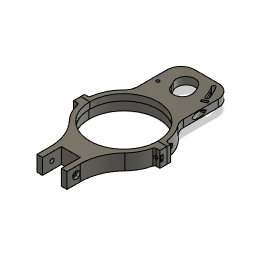
Generic Lens Mount and Focuser (Autodesk Fusion 360 design; units mm, degrees)
Autodesk Fusion 360 part; units mm, degrees
sketch "Sketch1" plane through (0, 0, 0) normal (0, 1, 0) x (1, 0, 0)
  circle A0 centre (0, 0) radius 37.25
  circle A1 centre (0, 0) radius 42.25
  line L0 (-37.25, 0) -> (37.25, 0) construction
  line L1 (-37.25, 0) -> (-42.25, 0)
  line L2 (37.25, 0) -> (42.25, 0)
  circle A2 centre (0.3022, 66.2) radius 21.95 construction
  circle A3 centre (-19.5912, 56.9235) radius 1.75
  arc A4 (11.2701, 65.1928) -> (6.5807, 75.2493) centre (-19.5912, 56.9235) ccw
  arc A5 (-8.0484, 60.0164) -> (11.2701, 65.1928) centre (1.6108, 62.6046) ccw
  arc A6 (-8.0484, 60.0164) -> (-9.8024, 63.7778) centre (-19.5912, 56.9235) ccw
  arc A7 (6.5807, 75.2493) -> (-9.8024, 63.7778) centre (-1.6108, 69.5135) ccw
  arc A8 (1.6108, 62.6046) -> (-1.6108, 69.5135) centre (-19.5912, 56.9235) ccw construction
  arc A9 (24.5033, 68.7386) -> (17.8031, 83.1073) centre (-19.5912, 56.9235) ccw
  arc A10 (21.1225, 67.8328) -> (24.5033, 68.7386) centre (22.8129, 68.2857) ccw
  arc A11 (21.1225, 67.8328) -> (14.936, 81.0998) centre (-19.5912, 56.9235) ccw
  arc A12 (17.8031, 83.1073) -> (14.936, 81.0998) centre (16.3695, 82.1035) ccw
  arc A13 (22.8129, 68.2857) -> (16.3695, 82.1035) centre (-19.5912, 56.9235) ccw construction
  line L3 (-19.5912, 56.9235) -> (16.3695, 82.1035) construction
  line L4 (-19.5912, 56.9235) -> (22.8129, 68.2857) construction
  line L5 (-25.3412, 33.8066) -> (-25.3412, 87.8535)
  line L6 (-25.3412, 87.8535) -> (30.5629, 87.8535)
  line L7 (0, 87.8535) -> (0, 0) construction
  circle A14 centre (0, 0) radius 38.25
  line L8 (16.3695, 82.1035) -> (22.8129, 68.2857)
  line L9 (-1.6108, 69.5135) -> (1.6108, 62.6046) construction
  line L10 (0, 66.0591) -> (1.6108, 62.6046)
  line L11 (-19.5912, 56.9235) -> (20.1957, 75.4765) construction
  line L12 (30.5629, 87.8535) -> (30.5629, 29.1714)
  line L13 (-42.25, 0) -> (-47.25, 0)
  line L14 (-47.25, 0) -> (-47.25, 4)
  line L15 (-47.25, 4) -> (-42.0602, 4)
  line L16 (47.25, 4) -> (42.0602, 4)
  line L17 (47.25, 0) -> (47.25, 4)
  line L18 (42.25, 0) -> (47.25, 0)
  line L19 (-47.25, 0) -> (-47.25, -7.85)
  line L20 (-47.25, -7.85) -> (-41.5143, -7.85)
  line L21 (47.25, 0) -> (47.25, -7.85)
  line L22 (47.25, -7.85) -> (41.5143, -7.85)
  line L23 (16.375, -38.9477) -> (16.375, -78.75)
  line L24 (16.375, -78.75) -> (10.375, -78.75)
  line L25 (10.375, -78.75) -> (10.375, -58)
  line L26 (10.375, -58) -> (-10.375, -58)
  line L27 (-10.375, -58) -> (-10.375, -78.75)
  line L28 (-10.375, -78.75) -> (-16.375, -78.75)
  line L29 (-16.375, -78.75) -> (-16.375, -38.9477)
  line L30 (0, 0) -> (0, -58)
  dimension "d1" = 74.5
  dimension "d2" = 5
  dimension "d3" = 43.9
  dimension "d4" = 3.5
  dimension "d5" = 10
  dimension "d7" = 1.75
  dimension "d8" = 20
  dimension "d11" = 5.75
  dimension "d14" = 76.5
  dimension "d26" = 65
  dimension "d28" = 5.75
  dimension "d29" = 7.75
  dimension "d57" = 5
  dimension "d58" = 4
  dimension "d59" = 7.85
  dimension "d94" = 66.2
  dimension "d99" = 6
  dimension "d100" = 6
  dimension "d101" = 20.75
  dimension "d102" = 20.75
  dimension "d123" = 58
  constraint coincident A0.centre A1.centre
  constraint coincident A0 L0.start
  constraint coincident A0 L0.end
  constraint coincident A0.centre L0
  constraint horizontal L0
  constraint coincident A1 L1.end
  constraint parallel L0 L1
  constraint coincident A1 L2.end
  constraint parallel L0 L2
  constraint coincident A2 A3.centre
  constraint tangent A4 A5
  constraint tangent A5 A6
  constraint tangent A6 A7
  constraint tangent A4 A7
  constraint coincident A3.centre A4.centre
  constraint coincident A2.centre A8
  constraint tangent A9 A10
  constraint tangent A10 A11
  constraint tangent A11 A12
  constraint tangent A9 A12
  constraint coincident A12.centre A13.end
  constraint coincident A10.centre A13.start
  constraint coincident A5.centre L4
  constraint coincident A7.centre L3
  constraint tangent A2 A13
  constraint coincident A1 L5.start
  constraint vertical L5
  constraint perpendicular L5 L6
  constraint vertical L7
  constraint concentric A0 A14
  constraint coincident A7.centre A8.end
  constraint coincident A5.centre A8.start
  constraint midpoint L9 L10.start
  constraint coincident L7 L10.start
  constraint midpoint A13 L11.end
  constraint coincident A2.centre L11
  constraint coincident A1 L12.end
  constraint perpendicular L6 L12
  constraint coincident L6 L7.start
  constraint parallel L1 L13
  constraint perpendicular L1 L14
  constraint coincident A1 L15.end
  constraint perpendicular L14 L15
  constraint symmetric L1.end L7 L2.end
  constraint symmetric L7 L13.end L17.start
  constraint symmetric L7 L14.end L16.start
  constraint symmetric L7 L15.end L16.end
  constraint perpendicular L13 L19
  constraint coincident A1 L20.end
  constraint perpendicular L19 L20
  constraint symmetric L7 L19.end L21.end
  constraint symmetric L7 L20.end L22.end
  constraint coincident A1 L23.start
  constraint vertical L23
  constraint perpendicular L23 L24
  constraint perpendicular L24 L25
  constraint perpendicular L25 L26
  constraint perpendicular L26 L27
  constraint perpendicular L27 L28
  constraint coincident A1 L29.end
  constraint perpendicular L28 L29
  constraint collinear L24 L28
  constraint midpoint L26 L30.end
  constraint vertical L30
  measures "d1" diameter of A0
  measures "d3" diameter of A2
  measures "d4" diameter of A3
  measures "d5" radius of A5
  measures "d7" radius of A10
  measures "d8" angle of L3 L4
  measures "d11" distance of A3.centre L5
  measures "d14" diameter of A14
  measures "d26" angle of L0 L8
  measures "d28" distance of A12.centre L6
  measures "d29" distance of A10.centre L12
  measures "d57" distance of L1.end L13.end
  measures "d58" distance of L13.end L14.end
  measures "d59" distance of L13.end L19.end
  measures "d94" vertical distance of A0.centre A2.centre
  measures "d99" distance of L23.end L24.end
  measures "d100" distance of L27.end L28.end
  measures "d101" distance of L25.end L26.end
  measures "d102" distance of L26.end L27.end
  measures "d123" distance of A0.centre L30.end
extrude "Extrude1" add sketch "Sketch1" along normal blind 7 contours A0 L1 L2 A14 | A1 L1 L2 A14 | A1 L16 L17 L18 | A1 L13 L14 L15 makes body 1
extrude "Extrude2" add sketch "Sketch1" against normal blind 10 contours A1 L1 L2 A14 | A1 L16 L17 L18 | A1 L13 L14 L15 bodies 1
extrude "Extrude3" add sketch "Sketch1" against normal blind 8 from surface at 7 contours A1 L5 L6 L12 bodies 1
extrude "Extrude4" add sketch "Sketch1" along normal blind 7 separate body contours A0 L2 A14 L30 | A0 L1 A14 L30 | A1 L2 A14 L30 | A1 L1 A14 L30 | A1 L18 L21 L22 | A1 L13 L19 L20 makes body 2
extrude "Extrude5" add sketch "Sketch1" against normal blind 10 contours A1 L2 A14 L30 | A1 L1 A14 L30 | A1 L18 L21 L22 | A1 L13 L19 L20 bodies 2
fillet "Fillet1" radius 15 2 edges at (-25.3412, 3, -87.8535) (30.5629, 3, -87.8535) on bodies 1
ref_plane "WorkPlane1" through (22.8129, 0, -68.2857) normal (0.422618, 0, 0.906308) x (0, 1, 0)
sketch "Sketch2" plane through (22.8129, 0, -68.2857) normal (0.422618, 0, 0.906308) x (0, 1, 0)
  line L0 (0, 0) -> (3, 0)
  circle A0 centre (3, 0) radius 1.75
  line L1 (4.7321, -3) -> (6.4641, 0) construction
  line L2 (6.4641, 0) -> (4.7321, 3) construction
  line L3 (4.7321, 3) -> (1.2679, 3)
  line L4 (1.2679, 3) -> (-0.4641, 0)
  line L5 (-0.4641, 0) -> (1.2679, -3)
  line L6 (1.2679, -3) -> (4.7321, -3)
  line L7 (3, 3) -> (7, 3)
  line L8 (7, 3) -> (7, -3)
  line L9 (3, -3) -> (7, -3)
  circle A1 centre (3, 0) radius 3.1
  point P0 (3, 0)
  dimension "d38" = 3.5
  dimension "d39" = 3
  dimension "d40" = 4
  dimension "d41" = 6.2
  dimension "d44" = 7
  constraint coincident L0.start origin
  constraint horizontal L0
  constraint coincident P0 L0.end
  constraint midpoint L3 L7.start
  constraint parallel L3 L7
  constraint perpendicular L3 L8
  constraint midpoint L6 L9.start
  constraint perpendicular L8 L9
  constraint concentric A0 A1
  constraint vertical L8
  measures "d38" diameter of A0
  measures "d39" distance of P0 L6
  measures "d40" distance of L9.start L8.end
  measures "d41" diameter of A1
  measures "d44" distance of L8 L0.start
extrude "Extrude6" cut sketch "Sketch2" along normal up to surface and the other way blind 15 contours A0 end surface through (30.5629, 7, -87.8535) normal (1, 0, 0) offset 0 bodies 1
extrude "Extrude7" cut sketch "Sketch2" along normal up to surface from surface at 10.5 contours L3 L4 L5 L6 L7 L9 A1 | L3 L7 A1 | L6 L9 A1 | L4 A1 | L5 A1 end surface through (30.5629, 7, -87.8535) normal (1, 0, 0) offset 0 bodies 1
extrude "Extrude8" cut sketch "Sketch2" along normal blind 2.65 from surface at 4 contours L3 L6 L7 L8 L9 A1 | L3 L4 L5 L6 L7 L9 A1 | L3 L4 A1 | L5 L6 A1 | L4 L5 A1 bodies 1
fillet "Fillet5" radius 2 2 edges at (-41.5143, -1.5, 7.85) (41.5143, -1.5, 7.85) on bodies 2
sketch "Sketch3" plane through (0, 0, -4) normal (0, 0, -1) x (-1, 0, 0)
  line L0 (47.25, -10) -> (47.25, 7)
  line L1 (47.25, 7) -> (42.0602, 7)
  line L2 (42.0602, 7) -> (42.0602, -10)
  line L3 (42.0602, -10) -> (47.25, -10)
  line L4 (47.25, -1.5) -> (43.25, -1.5) construction
  circle A0 centre (43.25, -1.5) radius 1.75
  circle A1 centre (43.25, -1.5) radius 3.1
  line L5 (44.9821, -4.5) -> (46.7141, -1.5) construction
  line L6 (46.7141, -1.5) -> (44.9821, 1.5) construction
  line L7 (44.9821, 1.5) -> (41.5179, 1.5)
  line L8 (41.5179, 1.5) -> (39.7859, -1.5)
  line L9 (39.7859, -1.5) -> (41.5179, -4.5)
  line L10 (41.5179, -4.5) -> (44.9821, -4.5)
  line L11 (44.9821, 1.5) -> (47.25, 1.5)
  line L12 (44.9821, -4.5) -> (47.25, -4.5)
  point P0 (43.25, -1.5)
  dimension "d60" = 4
  dimension "d61" = 3.5
  dimension "d62" = 6.2
  dimension "d63" = 3
  constraint midpoint L0 L4.start
  constraint perpendicular L2 L4
  constraint coincident P0 L4.end
  constraint concentric A0 A1
  constraint coincident L0 L11.end
  constraint perpendicular L0 L11
  constraint coincident L0 L12.end
  constraint perpendicular L0 L12
  constraint horizontal L10
  measures "d60" distance of L4.start P0
  measures "d61" diameter of A0
  measures "d62" diameter of A1
  measures "d63" distance of P0 L10
sketch "Sketch4" plane through (0, 0, -4) normal (0, 0, -1) x (-1, 0, 0)
  line L0 (-42.0602, -10) -> (-42.0602, 7)
  line L1 (-42.0602, 7) -> (-47.25, 7)
  line L2 (-47.25, 7) -> (-47.25, -10)
  line L3 (-47.25, -10) -> (-42.0602, -10)
  line L4 (-47.25, -1.5) -> (-43.25, -1.5) construction
  circle A0 centre (-43.25, -1.5) radius 1.75
  circle A1 centre (-43.25, -1.5) radius 3.1
  line L5 (-44.9821, 1.5) -> (-46.7141, -1.5) construction
  line L6 (-46.7141, -1.5) -> (-44.9821, -4.5) construction
  line L7 (-44.9821, -4.5) -> (-41.5179, -4.5)
  line L8 (-41.5179, -4.5) -> (-39.7859, -1.5)
  line L9 (-39.7859, -1.5) -> (-41.5179, 1.5)
  line L10 (-41.5179, 1.5) -> (-44.9821, 1.5)
  line L11 (-44.9821, 1.5) -> (-47.25, 1.5)
  line L12 (-44.9821, -4.5) -> (-47.25, -4.5)
  point P0 (-43.25, -1.5)
  dimension "d64" = 4
  dimension "d65" = 3.5
  dimension "d66" = 6.2
  dimension "d67" = 3
  constraint midpoint L2 L4.start
  constraint perpendicular L2 L4
  constraint coincident P0 L4.end
  constraint concentric A0 A1
  constraint coincident L2 L11.end
  constraint perpendicular L2 L11
  constraint coincident L2 L12.end
  constraint perpendicular L2 L12
  constraint horizontal L7
  measures "d64" distance of L4.start P0
  measures "d65" diameter of A0
  measures "d66" diameter of A1
  measures "d67" distance of P0 L10
extrude "Extrude11" cut sketch "Sketch3" along normal blind 14.076 and the other way through all contours L2 A0 | L2 A0 bodies 1 2
extrude "Extrude12" cut sketch "Sketch4" along normal blind 15.316 and the other way through all contours L0 A0 | L0 A0 bodies 1 2
extrude "Extrude13" cut sketch "Sketch3" along normal blind 36.08 contours L2 A0 A1 L7 L10 | A1 L10 | L2 A0 A1 L8 L9 | A1 L7 | A1 L9 | A1 L8 bodies 1
extrude "Extrude14" cut sketch "Sketch4" along normal blind 18.465 contours L0 A0 A1 L7 L10 | L0 A0 A1 L8 L9 | A1 L7 | A1 L8 | A1 L10 | A1 L9 bodies 1
extrude "Extrude15" cut sketch "Sketch3" along normal blind 2.65 from surface at -10.85 contours L0 A1 L7 L10 L11 L12 | L2 A1 L9 L10 | L2 A1 L10 | L2 A0 A1 L7 L10 | L2 A0 A1 L8 L9 | L2 A1 L7 | L2 A1 L7 L8 | A1 L8 L9 bodies 2
extrude "Extrude16" cut sketch "Sketch4" along normal blind 2.65 from surface at -10.85 contours L0 A1 L7 | L0 A1 L7 L8 | L0 A0 A1 L7 L10 | L0 A0 A1 L8 L9 | L2 A1 L7 L10 L11 L12 | A1 L8 L9 | L0 A1 L10 | L0 A1 L9 L10 bodies 2
fillet "Fillet2" radius 15 2 edges at (30.5629, 3, -29.1714) (-25.3412, 3, -33.8066) on bodies 1
fillet "Fillet3" radius 2 6 edges at (-42.0602, -7.1813, -4) (-42.0602, 4.1813, -4) (42.0602, 4.1813, -4) (42.0602, -7.1813, -4) (40.15, -1.5, -13.1545) (-40.15, -1.5, -13.1545) on bodies 1
fillet "Fillet4" radius 2 1 edges at (2.9234, -1, -42.1487) on bodies 1
extrude "Extrude17" add sketch "Sketch1" along normal blind 7 and the other way blind 10 contours A1 L26 L27 L28 L29 L30 | A1 L23 L24 L25 L26 L30 bodies 2
sketch "Sketch5" plane through (-10.375, 0, 0) normal (1, 0, 0) x (0, 0, -1)
  line L0 (-58, 7) -> (-78.75, 7)
  line L1 (-78.75, 7) -> (-78.75, -10)
  line L2 (-78.75, -10) -> (-58, -10)
  line L3 (-58, 7) -> (-78.75, -10) construction
  circle A0 centre (-68.375, -1.5) radius 2.25
  circle A1 centre (-68.375, -1.5) radius 4
  line L4 (-58, -10) -> (-58, 7)
  dimension "d109" = 4.5
  dimension "d110" = 8
  constraint coincident L0.start L3.start
  constraint coincident L1.end L2.start
  constraint midpoint L3 A0.centre
  constraint concentric A0 A1
  measures "d109" diameter of A0
  measures "d110" diameter of A1
fillet "Fillet6" radius 50 2 edges at (-16.375, -1.5, 38.9477) (16.375, -1.5, 38.9477) on bodies 2
extrude "Extrude18" cut sketch "Sketch5" along normal through all and the other way through all contours A0 bodies 2
extrude "Extrude19" cut sketch "Sketch5" against normal through all from surface at -3 contours A1 bodies 2
extrude "Extrude20" cut sketch "Sketch5" along normal through all from surface at 23.75 contours A1 bodies 2
equation "d1 = LensDiameter + 0.5 mm"
equation "d4 = M3Dim"
equation "d7 = M3Dim / 2"
equation "d8 = TensionRangeAngle"
equation "d11 = d4 / 2 + 4 mm"
equation "LensDiameter = 74 mm" comment "Set the overall diameter here"
equation "d14 = LensDiameter2 + 0.5 mm"
equation "d15 = LensDiameter1Length"
equation "d17 = -LensDiameter2Length"
equation "d19 = -MotorPlateThickness"
equation "d21 = LensDiameter1Length"
equation "d23 = -LensDiameter2Length"
equation "d26 = TensionTilt"
equation "d28 = d7 + 4 mm"
equation "d29 = d7 + 6 mm"
equation "TensionRangeAngle = 20 deg"
equation "TensionTilt = 65 deg"
equation "MotorPlateThickness = 8 mm"
equation "d39 = ( 5.5 / 2 ) * 1 mm + 0.25 mm"
equation "d40 = MotorPlateThickness / 2"
equation "d44 = LensDiameter1Length"
equation "M3Dim = 3.5 mm"
equation "d49 = M3Dim + 7 mm"
equation "d51 = M3Dim + 0.5 mm"
equation "LensDiameter2 = LensDiameter + 2 mm" comment "Set equal to LensDiameter1 if a smooth ID is needed."
equation "LensDiameter1Length = 7 mm"
equation "LensDiameter2Length = 10 mm"
equation "d61 = M3Dim"
equation "d63 = ( 5.5 / 2 ) * 1 mm + 0.25 mm"
equation "d65 = M3Dim"
equation "d67 = ( 5.5 / 2 ) * 1 mm + 0.25 mm"
equation "d94 = d1 / 2 + d2 + d3 / 2 + 2 mm"
equation "d100 = d99"
equation "d105 = LensDiameter1Length"
equation "d107 = LensDiameter2Length"
equation "d123 = LensHeightFromAlu"
equation "LensHeightFromAlu = 58 mm" comment "Increase this to raise the lens from the alu"
